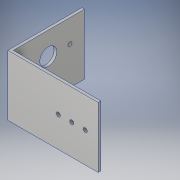
# Autodesk Inventor part: nhk16
Saved by Autodesk Inventor 2019 (Build 230136000, 136)
## iProperties
Created: 2022-02-15
Part Number: nhk16
Material: アルミニウム 6061
Document SubType Name: Sheet Metal
Designer: yuta
Density: 2.7 g/cm^3
Sheet Metal Rule: Default_mm
Appearance: アルミニウム - フラット
Author: yuta
Autodesk Inventor part; units mm, degrees
ref_plane "YZ Plane" through (0, 0, 0) normal (1, 0, 0) x (0, 1, 0)
ref_plane "XZ Plane" through (0, 0, 0) normal (0, 1, 0) x (-1, 0, 0)
ref_plane "XY Plane" through (0, 0, 0) normal (0, 0, 1) x (1, 0, 0)
sketch "スケッチ1" plane through (0, 0, 0) normal (0, 0, 1) x (1, 0, 0)
  line L0 (-10.5043, 6.5297) -> (54.4957, 6.5297)
  line L1 (54.4957, 6.5297) -> (54.4957, -38.4703)
  line L2 (54.4957, -38.4703) -> (-10.5043, -38.4703)
  line L3 (-10.5043, -38.4703) -> (-10.5043, 6.5297)
  point P0 (0, 0)
  dimension "d0" = 65
  dimension "d1" = 45
  constraints: 8 end point, 2 parallel, 1 horizontal, 1 perpendicular
  measures "d0" distance of L1.end L2.end
  measures "d1" distance of L0.end L1.end
extrude "押し出し1" add sketch "スケッチ1" along normal blind 2
sketch "スケッチ2" plane through (-10.5043, -38.4703, 0) normal (-1, 0, 0) x (0, 0, 1)
  line L0 (-53, 45) -> (2, 45)
  line L1 (2, 45) -> (2, 0)
  line L2 (2, 0) -> (-53, 0)
  line L3 (-53, 0) -> (-53, 45)
  point P0 (0, 38.4703)
  point P1 (2, 45)
  dimension "d4" = 55
  dimension "d5" = 45
  constraints: 8 end point, 2 parallel, 1 coincident, 1 horizontal, 1 perpendicular
  measures "d4" distance of L1.end L2.end
  measures "d5" distance of L0.end L1.end
extrude "押し出し2" add sketch "スケッチ2" along normal blind 2
sketch "スケッチ3" plane through (-12.5043, -38.4703, 0) normal (-1, 0, 0) x (0, 0, 1)
  circle A0 centre (-26, 28) radius 6.3
  line L0 (2, 45) -> (-53, 45) projected
  line L1 (-53, 0) -> (2, 0) projected
  line L2 (-53, 45) -> (-53, 0) projected
  point P0 (0, 38.4703)
  dimension "d8" = 12.6
  dimension "d10" = 28
  dimension "d11" = 27
  constraints: 1 centre point
  measures "d8" diameter of A0
  measures "d10" distance from line of L1 A0.centre
  measures "d11" distance from line of L2 A0.centre
extrude "押し出し3" cut sketch "スケッチ3" against normal blind 2
sketch "スケッチ4" plane through (-12.5043, -38.4703, 0) normal (-1, 0, 0) x (0, 0, 1)
  circle A0 centre (-42.1, 28) radius 1.5
  circle A1 centre (-26, 28) radius 6.3 projected
  line L0 (-53, 0) -> (2, 0) projected
  circle A2 centre (-9.9, 28) radius 1.5
  point P0 (0, 38.4703)
  dimension "d14" = 3
  dimension "d15" = 16.1
  dimension "d16" = 28
  dimension "d17" = 3
  dimension "d18" = 16.1
  constraints: 2 centre point
  measures "d14" diameter of A0
  measures "d15" distance of A0.centre A1.centre
  measures "d16" distance from line of L0 A0.centre
  measures "d17" diameter of A2
  measures "d18" distance of A1.centre A2.centre
hole "穴1" at (-12.5043, -10.4703, -42.1) at (-12.5043, -10.4703, -9.9) direction (1, 0, 0) diameter 3 depth 2
sketch "スケッチ5" plane through (0, 0, 2) normal (0, 0, 1) x (1, 0, 0)
  circle A0 centre (44.9957, -15.9703) radius 1.5
  line L0 (54.4957, -38.4703) -> (54.4957, 6.5297) projected
  line L1 (54.4957, 6.5297) -> (-12.5043, 6.5297) projected
  circle A1 centre (34.9957, -15.9703) radius 1.5
  circle A2 centre (24.9957, -15.9703) radius 1.5
  point P0 (0, 0)
  dimension "d26" = 3
  dimension "d27" = 9.5
  dimension "d28" = 22.5
  dimension "d29" = 3
  dimension "d30" = 3
  dimension "d31" = 10
  dimension "d32" = 10
  constraints: 3 centre point
  measures "d26" diameter of A0
  measures "d27" distance from line of L0 A0.centre
  measures "d28" distance from line of L1 A0.centre
  measures "d29" diameter of A1
  measures "d30" diameter of A2
  measures "d31" distance of A1.centre A0.centre
  measures "d32" distance of A2.centre A1.centre
hole "穴2" at (24.9957, -15.9703, 2) at (34.9957, -15.9703, 2) at (44.9957, -15.9703, 2) direction (0, 0, -1) diameter 3 depth 2
equation "\"BendRadius\" = Thickness"
equation "\"BendReliefWidth\" = Thickness"
equation "\"BendReliefDepth\" = 0.5 * Thickness"
equation "\"CornerReliefSize\" = 4 * Thickness"
equation "\"MinimumRemnant\" = 2 * Thickness"
equation "\"TransitionRadius\" = BendRadius"
equation "\"JacobiRadiusSize\" = BendRadius"
equation "\"GapSize\" = Thickness"
equation "\"Thickness\" = 0.5"
